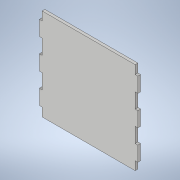
# Autodesk Inventor part: bottom-case
Saved by Autodesk Inventor 2020 (Build 240168000, 168)
## iProperties
Created: 2019-12-17
Part Number: bottom-case
Material: Generic
Document SubType Name: Modeling
Designer: fabfarm
Density: 1 g/cm^3
Appearance: Default
Author: fabfarm
Autodesk Inventor part; units mm, degrees
ref_plane "YZ Plane" through (0, 0, 0) normal (1, 0, 0) x (0, 1, 0)
ref_plane "XZ Plane" through (0, 0, 0) normal (0, 1, 0) x (-1, 0, 0)
ref_plane "XY Plane" through (0, 0, 0) normal (0, 0, 1) x (1, 0, 0)
sketch "Sketch1" plane through (0, 0, 0) normal (0, 0, 1) x (1, 0, 0)
  line L0 (330, -307.45) -> (-330, -307.45)
  line L1 (-330, -307.45) -> (-330, 307.45)
  line L2 (-330, 307.45) -> (330, 307.45)
  line L3 (330, 307.45) -> (330, -307.45)
  line L4 (330, -307.45) -> (-330, 307.45) construction
  line L5 (-330, -307.45) -> (330, 307.45) construction
  point P0 (0, 0)
  dimension "d0" = 614.9
  dimension "d1" = 660
  constraints: 12 end point, 2 midpoint, 2 parallel, 1 horizontal, 1 perpendicular
  measures "d0" distance of L2.end L0.start
  measures "d1" distance of L0.start L0.end
extrude "Extrusion1" add sketch "Sketch1" along normal blind 18.55
sketch "Sketch2" plane through (0, 0, 18.55) normal (0, 0, 1) x (1, 0, 0)
  line L0 (-330, 307.45) -> (-330, -307.45) projected
  line L1 (330, 307.45) -> (-330, 307.45) projected
  line L2 (-330, -307.45) -> (330, -307.45) projected
  line L3 (-330, -307.45) -> (-311.45, -307.45)
  line L4 (-311.45, -307.45) -> (-311.45, -250)
  line L5 (-311.45, -250) -> (-330, -250)
  line L6 (-330, -250) -> (-330, -307.45)
  line L7 (-330, 250) -> (-311.45, 250)
  line L8 (-311.45, 250) -> (-311.45, 307.45)
  line L9 (-311.45, 307.45) -> (-330, 307.45)
  line L10 (-330, 307.45) -> (-330, 250)
  line L11 (-330, 50) -> (-311.45, 50)
  line L12 (-311.45, 50) -> (-311.45, 150)
  line L13 (-311.45, 150) -> (-330, 150)
  line L14 (-330, 150) -> (-330, 50)
  line L15 (-330, -150) -> (-311.45, -150)
  line L16 (-311.45, -150) -> (-311.45, -50)
  line L17 (-311.45, -50) -> (-330, -50)
  line L18 (-330, -50) -> (-330, -150)
  point P0 (-330, -50)
  point P1 (-330, -250)
  dimension "d24" = 18.55
  dimension "d27" = 100
  dimension "d28" = 100
  dimension "d29" = 100
  dimension "d33" = 57.45
  dimension "d34" = 57.45
  dimension "d35" = 100
  constraints: 32 end point, 8 parallel, 5 point on line, 4 collinear, 4 horizontal, 4 perpendicular
  measures "d24" distance of L4.end L5.end
  measures "d27" distance of L15.end L16.end
  measures "d28" distance of L11.end L12.end
  measures "d29" distance between parallel lines of L11 L17
  measures "d33" distance of L3.end L4.end
  measures "d34" distance of L7.end L8.end
  measures "d35" distance between parallel lines of L15 L5
extrude "Extrusion2" cut sketch "Sketch2" against normal blind 18.55
mirror "Mirror1" about plane through (0, 0, 0) normal (1, 0, 0) of "Extrusion2"
sketch "Sketch3" plane through (0, 0, 18.55) normal (0, 0, 1) x (1, 0, 0)
  line L0 (-330, -307.45) -> (-330, 307.45) projected
  line L1 (-330, 305) -> (-311.45, 305) projected
  line L2 (-330, 307.45) -> (-311.45, 307.45)
  line L3 (-311.45, 307.45) -> (-311.45, 305)
  line L4 (-311.45, 305) -> (-330, 305)
  line L5 (-330, 305) -> (-330, 307.45)
  line L6 (311.45, 305) -> (330, 305) projected
  line L7 (-330, 307.45) -> (330, 307.45) projected
  line L8 (311.45, 305) -> (330, 305)
  line L9 (330, 305) -> (330, 307.45)
  line L10 (330, 307.45) -> (311.45, 307.45)
  line L11 (311.45, 307.45) -> (311.45, 305)
  point P0 (0, 0)
  constraints: 16 end point, 4 parallel, 2 horizontal, 2 perpendicular
extrude "Extrusion3" cut sketch "Sketch3" against normal blind 50
body "Solid1"
